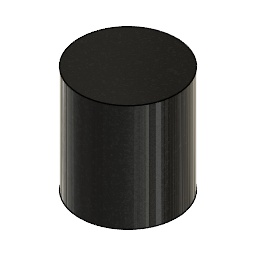
master_arm_complete (Autodesk Fusion 360 archive; units mm, degrees)
design "realknob"
part number: 2026-07-05-16-02-52-573
Autodesk Fusion 360 part; units mm, degrees
sketch "Sketch1" plane through (0, 0, 0) normal (0, 0, 1) x (1, 0, 0)
  circle A0 centre (0, 0) radius 7.25
  dimension "d1" = 14.5
  constraint coincident A0.centre origin
  measures "d1" diameter of A0
extrude "Extrude1" add sketch "Sketch1" along normal blind 16
shell "Shell1" thickness 1.5 removed faces 1 at (1.965, -0.3602, 0)
